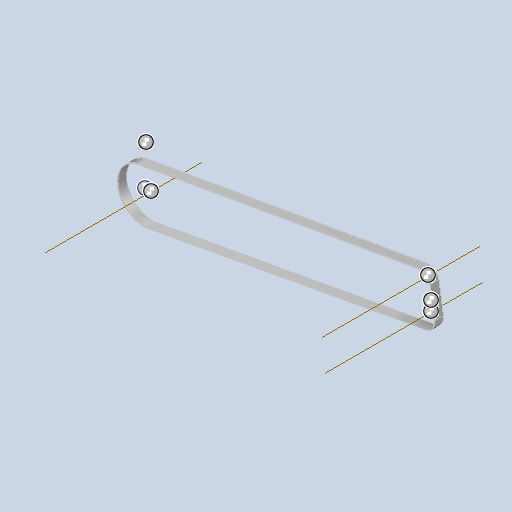
# Autodesk Inventor part: Pas synchroniczny
Saved by Autodesk Inventor 2023 (Build 270158000, 158)
## iProperties
CustomPartVersion: 1
Created: 2023-04-25
Part Number: Pas synchroniczny
Material: Rubber
Document SubType Name: Modeling
Designer: krzys
Density: 1 g/cm^3
Appearance: Rubber - Black - Version 1.1
Author: krzys
Autodesk Inventor part; units mm, degrees
ref_plane "YZ Plane" through (0, 0, 0) normal (1, 0, 0) x (0, 1, 0)
ref_plane "XZ Plane" through (0, 0, 0) normal (0, 1, 0) x (-1, 0, 0)
ref_plane "XY Plane" through (0, 0, 0) normal (0, 0, 1) x (1, 0, 0)
sketch "Ścieżka szkicu" plane through (0, 0, 0) normal (0, 0, 1) x (1, 0, 0)
  arc A0 (1.686486, 47.283213) -> (18.62403, -46.695093) centre (9.996476, 0.265443) ccw
  arc A1 (541.566622, 124.56248) -> (521.221373, 139.106582) centre (524.26837, 121.866733) ccw
  arc A2 (533.913231, 47.97344) -> (549.975522, 70.603679) centre (530.318417, 67.54033) ccw
  line L0 (533.913231, 47.97344) -> (18.62403, -46.695093)
  line L1 (1.686486, 47.283213) -> (521.221373, 139.106582)
  line L2 (541.566622, 124.56248) -> (549.975522, 70.603679)
  constraints: 6 end point, 6 point on circle, 3 centre point
ref_plane "Płaszczyzna przekroju poprzecznego" through (18.62403, -46.695093, 0) normal (0.9835392, 0.1806951, 0) x (0, 0, 1)
ref_plane "Płaszczyzna konstrukcyjna2" through (9.996476, 0.265443, 0) normal (-1, 0, 0) x (0, 0, 1)
ref_plane "Płaszczyzna konstrukcyjna3" through (524.26837, 121.866733, 0) normal (-0.9914046, -0.1308313, 0) x (0, 0, 1)
ref_plane "Płaszczyzna konstrukcyjna4" through (530.318417, 67.54033, 0) normal (0.0112485, 0.9999367, 0) x (0, 0, 1)
sketch "Przekrój poprzeczny" plane through (18.62403, -46.695093, 0) normal (0.9835392, 0.1806951, 0) x (0, 0, 1)
  line L0 (-8, 0.5) -> (8, 0.5)
  line L1 (8, 0.5) -> (8, -0.5)
  line L2 (8, -0.5) -> (-8, -0.5)
  line L3 (-8, -0.5) -> (-8, 0.5)
  line L4 (-8, 0) -> (8, 0) construction
  point P0 (0, 0)
  point P1 (0, 0)
  dimension "d0" = 16
  dimension "d4" = 0.5
  dimension "d5" = 0.5
  constraints: 10 end point, 3 midpoint, 2 parallel, 1 coincident, 1 horizontal, 1 perpendicular, 1 other
  measures "d0" distance between parallel lines of L1 L3
  measures "d4" distance between parallel lines of L2 L4
  measures "d5" distance between parallel lines of L4 L0
sweep "Pas" add profiles "Przekrój poprzeczny" path "Ścieżka szkicu" path curves L2 A2 L0 A0 L1 A1
equation "\"d0\" = da_B"
equation "\"d4\" = da_a"
equation "\"d5\" = da_a2"
equation "\"da_B\" = 16"
equation "\"da_pb\" = 5"
equation "\"da_L\" = 1315"
equation "\"da_a\" = 0.5"
equation "\"da_S\" = 2.65"
equation "\"da_Beta\" = 20deg"
equation "\"da_Ht\" = 1.2"
equation "\"da_H\" = 2.2"
equation "\"da_a2\" = 0.5"
body "Solid1"
